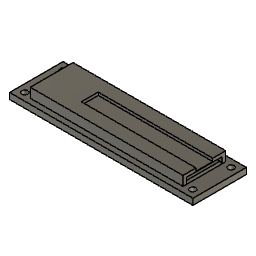
Suporte_comando_ (Autodesk Fusion 360 design; units mm, degrees)
Autodesk Fusion 360 part; units mm, degrees
sketch "Esboço1" plane through (0, 0, 0) normal (0, 0, 1) x (1, 0, 0)
  line L0 (0, 0) -> (120, 0)
  line L1 (120, 0) -> (120, 35)
  line L2 (120, 35) -> (0, 35)
  line L3 (0, 35) -> (0, 0)
  dimension "d1" = 120
  dimension "d2" = 35
  constraint horizontal L0
  constraint vertical L1
  constraint horizontal L2
  constraint vertical L3
  constraint coincident L0.start L3.end
  measures "d1" distance of L0.start L0.end
  measures "d2" distance of L0.start L2.end
extrude "Extrusão1" add sketch "Esboço1" along normal blind 4
sketch "Esboço2" plane through (0, 0, 4) normal (0, 0, 1) x (-1, 0, 0)
  line L0 (0, -35) -> (0, 0)
  line L1 (0, 0) -> (-120, 0)
  line L2 (-120, 0) -> (-120, -35)
  line L3 (-120, -35) -> (0, -35)
  line L4 (-10, -30) -> (-110, -30)
  line L5 (-110, -30) -> (-110, -5)
  line L6 (-110, -5) -> (-10, -5)
  line L7 (-10, -5) -> (-10, -30)
  point P0 (-5, -30)
  point P1 (-5, -5)
  point P2 (-115, -5)
  point P3 (-115, -30)
  constraint horizontal L4
  constraint vertical L5
  constraint horizontal L6
  constraint vertical L7
extrude "Extrusão2" add sketch "Esboço2" along normal blind 5 contours L4 L5 L6 L7
sketch "Esboço3" plane through (0, 0, 9) normal (0, 0, 1) x (-1, 0, 0)
  line L0 (-10, -5) -> (-110, -5)
  line L1 (-110, -5) -> (-110, -30)
  line L2 (-110, -30) -> (-10, -30)
  line L3 (-10, -30) -> (-10, -5)
sketch "Esboço4" plane through (110, 0, 0) normal (1, 0, 0) x (0, 1, 0)
  line L0 (5, 4) -> (30, 4)
  line L1 (30, 4) -> (30, 9)
  line L2 (30, 9) -> (5, 9)
  line L3 (5, 9) -> (5, 4)
  line L4 (5, 9) -> (5, 8)
  line L5 (30, 9) -> (30, 8)
  line L6 (5, 8) -> (30, 8)
  line L7 (6, 8) -> (6, 5)
  line L8 (6, 5) -> (29, 5)
  line L9 (29, 5) -> (29, 8)
  constraint coincident L2.end L3.start
  constraint coincident L3 L4.end
  constraint perpendicular L2 L4
  constraint coincident L1.end L2.start
  constraint coincident L1 L5.end
  constraint perpendicular L2 L5
  constraint perpendicular L1 L6
  constraint coincident L6 L7.start
  constraint perpendicular L6 L7
  constraint perpendicular L7 L8
  constraint coincident L6 L9.end
  constraint perpendicular L6 L9
extrude "Extrusão3" cut sketch "Esboço4" against normal blind 95 contours L6 L7 L8 L9
sketch "Esboço5" plane through (0, 0, 9) normal (0, 0, 1) x (1, 0, 0)
  line L0 (110, 30) -> (110, 23)
  line L1 (110, 5) -> (110, 12)
  line L2 (110, 23) -> (35, 23)
  line L3 (110, 12) -> (35, 12)
  line L4 (35, 12) -> (35, 23)
  line L5 (110, 23) -> (110, 12)
  dimension "d9" = 7
  dimension "d10" = 7
  constraint vertical L0
  constraint vertical L1
  constraint perpendicular L0 L2
  constraint perpendicular L1 L3
  constraint perpendicular L2 L4
  constraint perpendicular L3 L5
  measures "d9" distance of L0.start L0.end
  measures "d10" distance of L1.start L1.end
extrude "Extrusão4" cut sketch "Esboço5" against normal blind 5
sketch "Esboço6" plane through (0, 0, 4) normal (0, 0, 1) x (1, 0, 0)
extrude "Extrusão5" add 1 faces at (35, 15.6667, 4.3333) along direction (1, 0, 0) blind 75
sketch "Esboço7" plane through (110, 0, 0) normal (1, 0, 0) x (0, 1, 0)
  line L0 (5, 4) -> (30, 4)
  line L1 (30, 4) -> (30, 9)
  line L2 (30, 9) -> (23, 9)
  line L3 (23, 9) -> (23, 8)
  line L4 (23, 8) -> (29, 8)
  line L5 (29, 8) -> (29, 5)
  line L6 (29, 5) -> (6, 5)
  line L7 (6, 5) -> (6, 8)
  line L8 (6, 8) -> (12, 8)
  line L9 (12, 8) -> (12, 9)
  line L10 (12, 9) -> (5, 9)
  line L11 (5, 9) -> (5, 4)
  line L12 (6, 8) -> (29, 8)
  line L13 (29, 8) -> (29, 8.3)
  line L14 (29, 8.3) -> (6, 8.3)
  line L15 (6, 8.3) -> (6, 8)
  dimension "d15" = 0.3
  constraint horizontal L12
  constraint vertical L13
  constraint horizontal L14
  constraint vertical L15
  constraint coincident L7.end L8.start
  measures "d15" distance of L7.end L14.end
extrude "Extrusão6" add sketch "Esboço7" against normal blind 75 contours L3 L9 L12 L14
sketch "Esboço8" plane through (0, 0, 4) normal (0, 0, 1) x (1, 0, 0)
  circle A0 centre (5, 30) radius 2
  circle A1 centre (5, 5) radius 2
  circle A2 centre (115, 30) radius 2
  circle A3 centre (115, 5) radius 2
  dimension "d18" = 4
  dimension "d19" = 4
  dimension "d20" = 4
  dimension "d21" = 4
  measures "d18" diameter of A0
  measures "d19" diameter of A1
  measures "d20" diameter of A2
  measures "d21" diameter of A3
extrude "Extrusão7" cut sketch "Esboço8" against normal blind 20
sketch "Esboço9" plane through (10, 0, 0) normal (-1, 0, 0) x (0, -1, 0)
  line L0 (-30, 4) -> (-5, 4)
  line L1 (-5, 4) -> (-5, 9)
  line L2 (-5, 9) -> (-30, 9)
  line L3 (-30, 9) -> (-30, 4)
  line L4 (-30, 9) -> (-31.5, 9)
  line L5 (-31.5, 9) -> (-31.5, 4)
  line L6 (-31.5, 4) -> (-30, 4)
  line L7 (-30, 4) -> (-30, 9)
  line L8 (-5, 9) -> (-3.5, 9)
  line L9 (-3.5, 9) -> (-3.5, 4)
  line L10 (-3.5, 4) -> (-5, 4)
  line L11 (-5, 4) -> (-5, 9)
  dimension "d24" = 1.5
  dimension "d25" = 1.5
  dimension "d26" = 5
  constraint horizontal L4
  constraint vertical L5
  constraint horizontal L6
  constraint vertical L7
  constraint coincident L2.end L3.start
  constraint horizontal L8
  constraint vertical L9
  constraint horizontal L10
  constraint vertical L11
  constraint coincident L1.end L2.start
  measures "d24" distance of L2.end L4.end
  measures "d25" distance of L1.end L8.end
  measures "d26" distance of L1.end L0.end
extrude "Extrusão8" add sketch "Esboço9" against normal blind 100 contours L3 L4 L5 L6 L7 | L1 L8 L9 L10 L11
extrude "Extrusão9" add 1 faces at (18.3333, 19.3333, 9) along direction (0, 0, 1) blind 1.2
chamfer "Chanfro1" distance 1 angle 50 1 edges at (110, 17.5, 5) measured on face at (110, 4.3333, 7.4)
equation "d24 = ( 0.3 * 5 ) * 1 mm"
equation "d25 = ( 0.3 * 5 ) * 1 mm"
equation "d29 = ( 0.3 * 4 ) * 1 mm"
